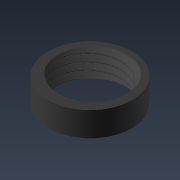
# Autodesk Inventor part: topPiece2
Saved by Autodesk Inventor 2022 (Build 260153000, 153)
## iProperties
Created: 2022-07-05
Part Number: topPiece2
Material: Generic
Document SubType Name: Modeling
Designer: User
Density: 1 g/cm^3
Appearance: Default
Author: User
## iProperties of the stored document topPiece2_3DPrint.ipt
Created: 2022-07-05
Part Number: topPiece2_3DPrint
Material: Generic
Document SubType Name: Modeling
Designer: User
Density: 1 g/cm^3
Appearance: Default
Author: User
Autodesk Inventor part; units mm, degrees
ref_plane "YZ Plane" through (0, 0, 0) normal (1, 0, 0) x (0, 1, 0)
ref_plane "XZ Plane" through (0, 0, 0) normal (0, 1, 0) x (-1, 0, 0)
ref_plane "XY Plane" through (0, 0, 0) normal (0, 0, 1) x (1, 0, 0)
sketch "Sketch1" plane through (0, 0, 0) normal (0, 1, 0) x (-1, 0, 0)
  circle A0 centre (0, 0) radius 15
  circle A1 centre (0, 0) radius 17
  dimension "d0" = 30
  dimension "d1" = 34
  constraints: 2 centre point, 2 coincident
  measures "d0" diameter of A0
  measures "d1" diameter of A1
extrude "Extrusion1" add sketch "Sketch1" along normal blind 10
thread "M22x3" size "M22x3" class "6H" standard "ANSI Metric M Profile" full length
sketch "Sketch5" plane through (0, 10, 0) normal (1, 0, 0) x (0, 0, 1)
  line L0 (15, 0) -> (15, 10)
  line L1 (15, 10) -> (12.7756, 10)
  line L2 (12.7756, 10) -> (12.7756, 0)
  line L3 (12.7756, 0) -> (15, 0)
  line L4 (0, -5.9256) -> (0, 12.6543) projected
  constraints: 8 end point
revolve "Revolution2" add sketch "Sketch5" angle 360 about axis through (0, 10, 0) along (0, -1, 0) separate body
sketch "Sketch4" plane through (0, 10, 15) normal (-1, 0, 0) x (0, -1, 0)
  line L0 (-1.7501, -0.1519) -> (-1.5001, -0.1519) construction
  line L1 (0.2499, -2.0728) -> (-0.0001, -2.5531) construction
  line L2 (-3.0001, -2.5531) -> (-3.2501, -2.0728) construction
  line L3 (-1.2501, -0.1519) -> (-1.5001, 0.3284) construction
  line L4 (-1.5001, 0.3284) -> (-1.7501, -0.1519) construction
  line L5 (-3.0001, -2.5531) -> (-2.7501, -2.0728) construction
  line L6 (-1.2501, -0.1519) -> (-0.2501, -2.0728)
  line L7 (-3.2501, -2.0728) -> (-2.7501, -2.0728) construction
  arc A0 (-3.2501, -2.0728) -> (-3.0001, -2.2246) centre (-3.0001, -1.9427) ccw construction
  line L8 (0.2499, -2.0728) -> (-0.2501, -2.0728) construction
  line L9 (-3.0001, -2.5531) -> (-3.0001, -2.0728) construction
  line L10 (-0.0001, -2.5531) -> (-0.0001, -2.0728) construction
  line L11 (-1.5001, 0.3284) -> (-1.5001, -0.0002) construction
  line L12 (-3.0001, -2.2246) -> (-0.0001, -2.2246)
  arc A1 (-3.0001, -2.2246) -> (-2.7501, -2.0728) centre (-3.0001, -1.9427) ccw
  line L13 (-0.2501, -2.0728) -> (-0.0001, -2.5531) construction
  line L14 (-2.7501, -2.0728) -> (-1.7501, -0.1519)
  line L15 (-0.0001, -0.0002) -> (-0.0001, 0.0177)
  line L16 (-0.0001, 0.0177) -> (-0.0001, -0.0002)
  line L17 (-0.0001, -0.0002) -> (0.0334, -0.0002)
  arc A2 (-0.2501, -2.0728) -> (-0.0001, -2.2246) centre (-0.0001, -1.9427) ccw
  arc A3 (-0.0001, -2.2246) -> (0.2499, -2.0728) centre (-0.0001, -1.9427) ccw construction
  arc A4 (-1.5001, -0.0002) -> (-1.7501, -0.1519) centre (-1.5001, -0.282) ccw
  arc A5 (-1.2501, -0.1519) -> (-1.5001, -0.0002) centre (-1.5001, -0.282) ccw
  line L18 (-1.5001, -0.0002) -> (-1.5001, -0.1519) construction
  line L19 (-1.5001, -0.1519) -> (-1.2501, -0.1519) construction
  dimension "d24" = 55
  dimension "d25" = 0.4803
  dimension "d26" = 0.4803
  dimension "Sketch4_ThreadOffset" = 0
  dimension "Sketch4_MajorRadius" = 2.2244
  dimension "d29" = 3
  dimension "Sketch4_MinorRadius" = 0
  constraints: 40 end point, 12 point on circle, 10 parallel, 8 tangent, 6 centre point, 6 collinear, 2 midpoint, 2 point on line, 1 horizontal, 1 perpendicular, 3 other
  measures "d24" angle of L6 L14
  measures "d25" distance of L3.end L0.end
  measures "d26" distance of L1.end L10.end
  measures "Sketch4_ThreadOffset" distance between parallel lines of L15 L10
  measures "Sketch4_MajorRadius" distance from line of L12 L15.start
  measures "d29" distance from line of L1.end L9
  measures "Sketch4_MinorRadius" distance edge to line of A5 L17
coil "Coil2" sketch "Sketch4" operation cut axis through (0, 10, 0) along (0, -1, 0) pitch 3.003 turns 5.328005 hand right bodies 2
equation "\"d24\" = d31"
equation "\"d25\" = 0.160083 * Sketch4_Pitch"
equation "\"d26\" = 0.160083 * Sketch4_Pitch"
equation "\"d29\" = Sketch4_Pitch"
equation "\"d13\" = 55deg"
equation "\"Sketch2_Pitch\" = 2"
equation "\"d31\" = 55deg"
equation "\"Sketch4_Pitch\" = 3"
body "Solid1"
body "Solid3"
